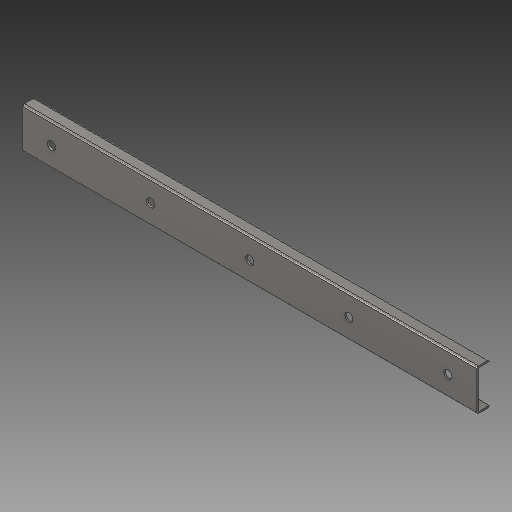
# Autodesk Inventor part: support1
Saved by Autodesk Inventor 2019 (Build 230136000, 136)
## iProperties
Created: 2019-02-23
Part Number: support1
Material: Stainless Steel
Document SubType Name: Modeling
Designer: gaincarlo
Density: 8 g/cm^3
Appearance: Semi-Polished
Author: gaincarlo
Autodesk Inventor part; units mm, degrees
ref_plane "YZ Plane" through (0, 0, 0) normal (1, 0, 0) x (0, 1, 0)
ref_plane "XZ Plane" through (0, 0, 0) normal (0, 1, 0) x (-1, 0, 0)
ref_plane "Work Plane1" through (0, 0, 0) normal (0, 0, 1) x (1, 0, 0)
sketch "Sketch1" plane through (0, 0, 0) normal (0, 0, 1) x (1, 0, 0)
  line L0 (195.6597, 725) -> (745.6597, 725)
  line L1 (745.6597, 725) -> (745.6597, 775)
  line L2 (745.6597, 775) -> (195.6597, 775)
  line L3 (195.6597, 775) -> (195.6597, 725)
  line L4 (164.0316, 10) -> (164.0316, 1490) projected
  line L5 (777.2877, 10) -> (164.0316, 10) projected
  line L6 (470.6597, 10) -> (470.6597, 1506) construction
  line L7 (164.0316, 750) -> (680, 750) construction
  point P0 (0, 0)
  point P1 (470.6597, 725)
  point P2 (195.6597, 750)
  dimension "d0" = 550
  dimension "d1" = 50
  constraints: 12 end point, 4 midpoint, 2 horizontal, 2 parallel, 2 point on line, 1 perpendicular, 1 vertical
  measures "d0" distance of L2.end L1.end
  measures "d1" distance of L1.end L0.end
extrude "Extrusion1" add sketch "Sketch1" along normal blind 15
sketch "Sketch2" plane through (195.6597, 725, 0) normal (-1, 0, 0) x (0, 0, 1)
  line L0 (15, 0) -> (0, 0) projected
  line L1 (0, 0) -> (0, 50) projected
  line L2 (0, 50) -> (15, 50) projected
  line L3 (15, 50) -> (15, 0) projected
  line L4 (12, 48) -> (0, 48)
  line L5 (0, 2) -> (12, 2)
  line L6 (13, 3) -> (13, 47)
  arc A0 (13, 47) -> (12, 48) centre (12, 47) ccw
  arc A1 (12, 2) -> (13, 3) centre (12, 3) ccw
  point P0 (0, -725)
  dimension "d5" = 2
  constraints: 6 end point, 4 point on circle, 4 tangent, 2 centre point, 2 point on line, 1 equal radius
  measures "d5" distance between parallel lines of L2 L4
extrude "Extrusion2" cut sketch "Sketch2" against normal through all contours L1 L4 A0 L6 A1 L5
fillet "Fillet1" radius 2 4 edges at (470.6597, 775, 15) (470.6597, 775, 0) (470.6597, 725, 0) (470.6597, 725, 15)
sketch "Sketch3" plane through (0, 0, 15) normal (0, 0, 1) x (1, 0, 0)
  line L0 (195.6597, 727) -> (745.6597, 727) construction
  line L1 (745.6597, 773) -> (745.6597, 727) construction
  line L2 (745.6597, 773) -> (195.6597, 773) construction
  line L3 (195.6597, 727) -> (195.6597, 773) construction
  line L4 (195.6597, 772) -> (745.6597, 772) projected
  line L5 (470.6597, 772) -> (470.6597, 727) construction
  circle A0 centre (470.6597, 749.5) radius 5
  point P0 (0, 0)
  dimension "d10" = 10
  constraints: 3 midpoint, 2 end point, 1 centre point, 1 vertical
  measures "d10" diameter of A0
extrude "Extrusion3" cut sketch "Sketch3" against normal up to next
pattern_linear "Rectangular Pattern1" count 5 spacing 120 along (1, 0, 0) of "Extrusion3" first direction both ways yes
body "Solid1"
